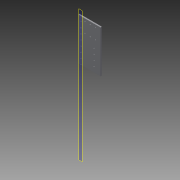
# Autodesk Inventor part: Aluminum Final
Saved by Autodesk Inventor 2015 (Build 190159000, 159)
## iProperties
Created: 2015-01-28
Part Number: Aluminum Final
Material: Generic
Document SubType Name: Modeling
Designer: jhirshland1
Mass: 136.068 g
Surface Area: 487.177 cm^2
Volume: 136.068 cm^3
Density: 1 g/cm^3
Appearance: Default
Author: jhirshland1
Autodesk Inventor part; units mm, degrees
ref_plane "YZ Plane" through (0, 0, 0) normal (1, 0, 0) x (0, 1, 0)
ref_plane "XZ Plane" through (0, 0, 0) normal (0, 1, 0) x (-1, 0, 0)
ref_plane "XY Plane" through (0, 0, 0) normal (0, 0, 1) x (1, 0, 0)
ref_plane "Work Plane1" through (-113.4922, 95.6302, 200.3599) normal (-0.0001, 0, -1) x (0, -1, 0)
sketch "Sketch1" plane through (-113.4922, 95.6302, 200.3599) normal (-0.0001, 0, -1) x (0, -1, 0)
  line L0 (212.1169, -104.14) -> (330.2269, -104.14) projected
  line L1 (117.2921, 3.175) -> (320.7139, 3.175)
  line L2 (320.7139, 3.175) -> (320.7139, -104.14)
  line L3 (320.7139, -104.14) -> (117.2921, -104.14)
  line L4 (117.2921, -104.14) -> (117.2921, 3.175)
  circle A0 centre (129.9921, -79.375) radius 2.667 projected
  circle A1 centre (129.9921, -53.975) radius 2.667 projected
  circle A2 centre (129.9921, -28.575) radius 2.667 projected
  circle A3 centre (139.7, -9.525) radius 2.667 projected
  circle A4 centre (165.1, -9.525) radius 2.667 projected
  circle A5 centre (180.3669, -28.575) radius 2.667 projected
  circle A6 centre (180.3669, -53.975) radius 2.667 projected
  circle A7 centre (180.3669, -79.375) radius 2.667 projected
  circle A8 centre (292.1, -9.525) radius 2.667 projected
  circle A9 centre (317.5, -9.525) radius 2.667 projected
  circle A10 centre (266.7, -9.525) radius 2.667 projected
  circle A11 centre (241.3, -9.525) radius 2.667 projected
  circle A12 centre (215.9, -9.525) radius 2.667 projected
  circle A13 centre (190.5, -9.525) radius 2.667 projected
  circle A14 centre (295.3019, -72.39) radius 2.667 projected
  circle A15 centre (269.9019, -72.39) radius 2.667 projected
  circle A16 centre (244.5019, -72.39) radius 2.667 projected
  circle A17 centre (219.1019, -72.39) radius 2.667 projected
  point P0 (95.6298, -113.5035)
  constraints: 8 end point, 2 parallel, 1 horizontal, 1 perpendicular, 1 point on line, 1 other
extrude "Extrusion1" add sketch "Sketch1" along normal blind 6.35
body "Solid1"
